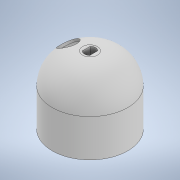
# Autodesk Inventor part: acoplamento joystick
Saved by Autodesk Inventor 2022 (Build 260153000, 153)
## iProperties
Created: 2024-04-24
Part Number: acoplamento joystick
Material: Generic
Document SubType Name: Modeling
Designer: admin
Density: 1 g/cm^3
Appearance: Default
Author: admin
Autodesk Inventor part; units mm, degrees
ref_plane "YZ Plane" through (0, 0, 0) normal (1, 0, 0) x (0, 1, 0)
ref_plane "XZ Plane" through (0, 0, 0) normal (0, 1, 0) x (-1, 0, 0)
ref_plane "XY Plane" through (0, 0, 0) normal (0, 0, 1) x (1, 0, 0)
sketch "Sketch1" plane through (0, 0, 0) normal (0, 1, 0) x (-1, 0, 0)
  circle A0 centre (0, 0) radius 15.6
  dimension "d0" = 31.2
  constraints: 1 centre point, 1 coincident
  measures "d0" diameter of A0
extrude "Extrusion1" add sketch "Sketch1" along normal blind 28
fillet "Fillet1" radius 12.5 1 edges at (15.6, 28, 0)
sketch "Sketch2" plane through (0, 0, 0) normal (0, -1, 0) x (1, 0, 0)
  circle A0 centre (0, 0) radius 14.75
  dimension "d4" = 29.5
  constraints: 1 centre point, 1 coincident
  measures "d4" diameter of A0
extrude "Extrusion2" cut sketch "Sketch2" against normal blind 8.3
shell "Shell2" thickness 0.85 removed faces 0
sketch "Sketch5" plane through (0, 8.3, 0) normal (0, -1, 0) x (1, 0, 0)
  circle A0 centre (0, 0) radius 3.1 projected
  circle A1 centre (0, 0) radius 14.75
  dimension "d14" = 29.5
  constraints: 1 centre point, 1 coincident
  measures "d14" diameter of A1
extrude "Extrusion5" cut sketch "Sketch5" against normal blind 2.2 contours A0 | A1
sketch "Sketch6" plane through (0, 27.15, 0) normal (0, -1, 0) x (1, 0, 0)
  circle A0 centre (0, 0) radius 3.1 projected
  circle A1 centre (0, 0) radius 3
  dimension "d17" = 6
  constraints: 1 centre point, 1 coincident
  measures "d17" diameter of A1
extrude "Extrusion6" add sketch "Sketch6" along normal blind 6 contours A1
sketch "Sketch7" plane through (0, 28, 0) normal (0, 1, 0) x (1, 0, 0)
  circle A0 centre (0, 0) radius 2.3
  line L0 (-1.5775, 1.6738) -> (1.5775, 1.6738)
  line L1 (1.5775, 1.6738) -> (1.5775, -1.6738)
  line L2 (1.5775, -1.6738) -> (-1.5775, -1.6738)
  line L3 (-1.5775, -1.6738) -> (-1.5775, 1.6738)
  line L4 (-1.5775, 1.6738) -> (1.5775, -1.6738) construction
  line L5 (1.5775, 1.6738) -> (-1.5775, -1.6738) construction
  dimension "d20" = 4.6
  constraints: 12 end point, 2 midpoint, 2 parallel, 1 coincident, 1 horizontal, 1 perpendicular, 3 other
extrude "Extrusion7" cut sketch "Sketch7" against normal blind 5 contours L0 A0 | L1 L2 L3 L0 | A0 L2
sketch "Sketch9" plane through (0, 28, 0) normal (0, 1, 0) x (1, 0, 0)
  circle A0 centre (0, 0) radius 3.1 projected
  line L0 (0, 0) -> (-9, 0)
  circle A1 centre (-9, 0) radius 3.5
  dimension "d34" = 9
  dimension "d35" = 7
  constraints: 2 end point, 1 centre point, 1 coincident, 1 horizontal
  measures "d34" distance of L0.start L0.end
  measures "d35" diameter of A1
extrude "Extrusion9" cut sketch "Sketch9" against normal blind 10 contours A1
sketch "Sketch10" plane through (0, 0, 0) normal (0, -1, 0) x (1, 0, 0)
  circle A0 centre (0, 0) radius 14.75 projected
  line L0 (0, -14.75) -> (-2, -14.75)
  line L1 (-2, -14.75) -> (-2, -13.75)
  line L2 (-2, -13.75) -> (0, -13.75)
  line L3 (0, -14.75) -> (2, -14.75)
  line L4 (2, -14.75) -> (2, -13.75)
  line L5 (2, -13.75) -> (0, -13.75)
  line L6 (11.7739, -9.1071) -> (10.9078, -8.6071)
  line L7 (12.7739, -7.375) -> (11.7739, -9.1071)
  line L8 (12.7739, -7.375) -> (13.7739, -5.6429)
  line L9 (13.7739, -5.6429) -> (12.9078, -5.1429)
  line L10 (12.9078, -5.1429) -> (11.9078, -6.875)
  line L11 (10.9078, -8.6071) -> (11.9078, -6.875)
  line L12 (13.7739, 5.6429) -> (12.9078, 5.1429)
  line L13 (12.7739, 7.375) -> (13.7739, 5.6429)
  line L14 (12.7739, 7.375) -> (11.7739, 9.1071)
  line L15 (11.7739, 9.1071) -> (10.9078, 8.6071)
  line L16 (10.9078, 8.6071) -> (11.9078, 6.875)
  line L17 (12.9078, 5.1429) -> (11.9078, 6.875)
  line L18 (2, 14.75) -> (2, 13.75)
  line L19 (0, 14.75) -> (2, 14.75)
  line L20 (0, 14.75) -> (-2, 14.75)
  line L21 (-2, 14.75) -> (-2, 13.75)
  line L22 (-2, 13.75) -> (0, 13.75)
  line L23 (2, 13.75) -> (0, 13.75)
  line L24 (-11.7739, 9.1071) -> (-10.9078, 8.6071)
  line L25 (-12.7739, 7.375) -> (-11.7739, 9.1071)
  line L26 (-12.7739, 7.375) -> (-13.7739, 5.6429)
  line L27 (-13.7739, 5.6429) -> (-12.9078, 5.1429)
  line L28 (-12.9078, 5.1429) -> (-11.9078, 6.875)
  line L29 (-10.9078, 8.6071) -> (-11.9078, 6.875)
  line L30 (-13.7739, -5.6429) -> (-12.9078, -5.1429)
  line L31 (-12.7739, -7.375) -> (-13.7739, -5.6429)
  line L32 (-12.7739, -7.375) -> (-11.7739, -9.1071)
  line L33 (-11.7739, -9.1071) -> (-10.9078, -8.6071)
  line L34 (-10.9078, -8.6071) -> (-11.9078, -6.875)
  line L35 (-12.9078, -5.1429) -> (-11.9078, -6.875)
  point P0 (-11.6559, 9.0389)
  point P1 (-13.6559, 5.5748)
  point P2 (0, 13.75)
  point P3 (2, 14.6138)
  point P4 (-2, 14.6138)
  point P5 (13.6559, 5.5748)
  point P6 (11.6559, 9.0389)
  point P7 (11.6559, -9.0389)
  point P8 (13.6559, -5.5748)
  point P9 (-2, -14.6138)
  point P10 (2, -14.6138)
  point P11 (-13.6559, -5.5748)
  point P12 (-11.6559, -9.0389)
  dimension "d36" = 2
  dimension "d37" = 1
  dimension "d38" = 2
  dimension "d41" = 360
  constraints: 72 end point, 6 point on line, 2 horizontal, 2 parallel, 2 perpendicular, 81 other
  measures "d36" distance of L1.end L2.end
  measures "d37" distance of L0.end L1.end
  measures "d38" distance of L5.end L4.end
extrude "Extrusion10" add sketch "Sketch10" against normal blind 1 contours L12 L17 L16 L15 A0 | A0 L6 L11 L10 L9 | L18 L23 L22 L21 A0 | A0 L1 L2 L5 L4 | L24 L29 L28 L27 A0 | A0 L30 L35 L34 L33
body "Solid1"
